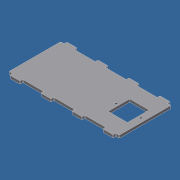
# Autodesk Inventor part: P1704_V2_ParoiLarge
Saved by Autodesk Inventor 2015 SP2 (Build 190223200, 223)
## iProperties
Created: 2017-02-08
Part Number: P1704_V2_ParoiLarge
Project: Nom Projet
Material: .
Description: Nom pièce
Document SubType Name: Modeling
Designer: Boris.GAUDARD
Authority: brut Ø
Density: 0.001 g/cm^3
Appearance: Par défaut
Material number: ---
Author: Boris.GAUDARD
Autodesk Inventor part; units mm, degrees
ref_plane "Plan YZ" through (0, 0, 0) normal (1, 0, 0) x (0, 1, 0)
ref_plane "Plan XZ" through (0, 0, 0) normal (0, 1, 0) x (-1, 0, 0)
ref_plane "Plan XY" through (0, 0, 0) normal (0, 0, 1) x (1, 0, 0)
sketch "Esquisse1" plane through (0, 0, 0) normal (0, 0, 1) x (1, 0, 0)
  line L0 (0, -58.1) -> (0, 58.1) construction
  line L1 (-112, 0) -> (112, 0) construction
  line L2 (-75, 37.5) -> (-75, 41.5)
  line L3 (-75, 41.5) -> (-60, 41.5)
  line L4 (-60, 41.5) -> (-60, 37.5)
  line L5 (-30, 37.5) -> (-30, 41.5)
  line L6 (-30, 41.5) -> (-15, 41.5)
  line L7 (-15, 41.5) -> (-15, 37.5)
  line L8 (15, 37.5) -> (15, 41.5)
  line L9 (15, 41.5) -> (30, 41.5)
  line L10 (30, 41.5) -> (30, 37.5)
  line L11 (60, 37.5) -> (60, 41.5)
  line L12 (60, 41.5) -> (75, 41.5)
  line L13 (75, 41.5) -> (75, 37.5)
  line L14 (-60, 37.5) -> (-30, 37.5)
  line L15 (-15, 37.5) -> (15, 37.5)
  line L16 (30, 37.5) -> (60, 37.5)
  line L17 (-75, 37.5) -> (-80, 37.5)
  line L18 (75, 37.5) -> (80, 37.5)
  line L19 (-75, -37.5) -> (-75, -41.5)
  line L20 (-75, -41.5) -> (-60, -41.5)
  line L21 (-60, -41.5) -> (-60, -37.5)
  line L22 (-30, -37.5) -> (-30, -41.5)
  line L23 (-30, -41.5) -> (-15, -41.5)
  line L24 (-15, -41.5) -> (-15, -37.5)
  line L25 (15, -37.5) -> (15, -41.5)
  line L26 (15, -41.5) -> (30, -41.5)
  line L27 (30, -41.5) -> (30, -37.5)
  line L28 (60, -37.5) -> (60, -41.5)
  line L29 (60, -41.5) -> (75, -41.5)
  line L30 (75, -41.5) -> (75, -37.5)
  line L31 (-60, -37.5) -> (-30, -37.5)
  line L32 (-15, -37.5) -> (15, -37.5)
  line L33 (30, -37.5) -> (60, -37.5)
  line L34 (-75, -37.5) -> (-80, -37.5)
  line L35 (75, -37.5) -> (80, -37.5)
  line L36 (80, -37.5) -> (80, 37.5)
  line L37 (-80, 37.5) -> (-80, -37.5)
  dimension "d2" = 15
  dimension "d8" = 45
  dimension "d13" = 5
  dimension "d14" = 5
  dimension "d15" = 75
  dimension "d16" = 4
  dimension "d17" = 160
  constraints: 72 end point, 18 symmetric about line, 4 horizontal, 2 perpendicular, 2 point on line, 2 vertical, 1 collinear, 22 other
  measures "d2" distance between parallel lines of L4 L2
  measures "d8" distance of L2.start L5.start
  measures "d13" distance of L13.end L18.end
  measures "d14" distance of L2.start L17.end
  measures "d15" distance between parallel lines of L33 L16
  measures "d16" distance between parallel lines of L14 L3
  measures "d17" distance between parallel lines of L36 L37
extrude "Extrusion1" add sketch "Esquisse1" along normal blind 4
sketch "Esquisse6" plane through (0, 0, 4) normal (0, 0, 1) x (1, 0, 0)
  line L0 (0, -58.1) -> (0, 58.1) construction
  line L1 (-112, 0) -> (112, 0) construction
  point P0 (0, 0)
  point P1 (-75, 37.5)
  point P2 (-60, 37.5)
  point P3 (-30, 37.5)
  point P4 (-15, 37.5)
  point P5 (15, 37.5)
  point P6 (75, 37.5)
  point P7 (30, 37.5)
  point P8 (60, 37.5)
  point P9 (-75, -37.5)
  point P10 (-60, -37.5)
  point P11 (-30, -37.5)
  point P12 (-15, -37.5)
  point P13 (15, -37.5)
  point P14 (75, -37.5)
  point P15 (30, -37.5)
  point P16 (60, -37.5)
  constraints: 8 symmetric about line
hole "Perçage1" at (-75, 37.5, 4) at (-60, 37.5, 4) at (-30, 37.5, 4) at (-15, 37.5, 4) at (15, 37.5, 4) at (75, 37.5, 4) at (30, 37.5, 4) at (60, 37.5, 4) at (60, -37.5, 4) at (30, -37.5, 4) at (75, -37.5, 4) at (15, -37.5, 4) at (-15, -37.5, 4) at (-30, -37.5, 4) at (-60, -37.5, 4) at (-75, -37.5, 4) direction (0, 0, -1) diameter 1 end through all
chamfer "Chanfrein1" distance 1 angle 45 16 edges at (75, 41.5, 2) (60, 41.5, 2) (15, 41.5, 2) (-30, 41.5, 2) (-75, 41.5, 2) (30, 41.5, 2) (-15, 41.5, 2) (-60, 41.5, 2) (-60, -41.5, 2) (-15, -41.5, 2) (30, -41.5, 2) (75, -41.5, 2) (60, -41.5, 2) (-75, -41.5, 2) (-30, -41.5, 2) (15, -41.5, 2)
chamfer "Chanfrein2" distance 1 angle 45 4 edges at (-80, 37.5, 2) (-80, -37.5, 2) (80, -37.5, 2) (80, 37.5, 2)
sketch "Esquisse7" plane through (0, 0, 4) normal (0, 0, 1) x (1, 0, 0)
  line L0 (42, 15.6) -> (70, 15.6)
  line L1 (70, 15.6) -> (70, -15.6)
  line L2 (70, -15.6) -> (42, -15.6)
  line L3 (42, -15.6) -> (42, 15.6)
  line L4 (-112, 0) -> (112, 0) construction
  line L5 (0, -58.1) -> (0, 58.1) construction
  line L6 (80, -36.5) -> (80, 36.5) construction
  point P0 (0, 0)
  dimension "d33" = 31.2
  dimension "d34" = 28
  dimension "d36" = 10
  constraints: 8 end point, 2 parallel, 1 horizontal, 1 perpendicular, 1 other
  measures "d33" distance between parallel lines of L2 L0
  measures "d34" distance between parallel lines of L3 L1
  measures "d36" distance between parallel lines of L6 L1
extrude "Extrusion2" cut sketch "Esquisse7" against normal blind 10
sketch "Esquisse8" plane through (0, 0, 4) normal (0, 0, 1) x (1, 0, 0)
  line L0 (-112, 0) -> (112, 0) construction
  line L1 (80, -36.5) -> (80, 36.5) construction
  point P0 (0, 0)
  point P1 (74, 0)
  point P2 (38, 0)
  dimension "d39" = 36
  dimension "d40" = 6
  constraints: 2 point on line
  measures "d39" distance of point (38, 0) point (74, 0)
  measures "d40" distance from line of L1 point (74, 0)
hole "Perçage2" at (74, 0, 4) at (38, 0, 4) direction (0, 0, -1) diameter 3.2 end through all clearance for "Vis à tête plate fraisée ISO 2009/7046" size "M3" standard "ISO"
